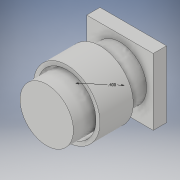
# Autodesk Inventor part: Ring Tolerance Test 6
Saved by Autodesk Inventor 2018 (Build 220112000, 112)
## iProperties
Created: 2019-08-26
Part Number: Ring Tolerance Test 6
Material: Generic
Document SubType Name: Modeling
Designer: 871357
Density: 1 g/cm^3
Appearance: Default
Author: 871357
Autodesk Inventor part; units mm, degrees
ref_plane "YZ Plane" through (0, 0, 0) normal (1, 0, 0) x (0, 1, 0)
ref_plane "XZ Plane" through (0, 0, 0) normal (0, 1, 0) x (-1, 0, 0)
ref_plane "XY Plane" through (0, 0, 0) normal (0, 0, 1) x (1, 0, 0)
sketch "Sketch1" plane through (0, 0, 0) normal (0, 0, 1) x (1, 0, 0)
  circle A0 centre (0, 0) radius 5.08
  dimension "d0" = 10.16
  constraints: 1 centre point, 1 coincident
  measures "d0" diameter of A0
extrude "Extrusion1" add sketch "Sketch1" along normal blind 10.16
ref_plane "Work Plane1" through (0, 0, 5.08) normal (0, 0, -1) x (-1, 0, 0)
sketch "Sketch4" plane through (0, 0, 0) normal (0, 0, -1) x (-1, 0, 0)
  circle A0 centre (0, 0) radius 5.588
  circle A1 centre (0, 0) radius 6.35
  dimension "d13" = 11.176
  dimension "d14" = 12.7
  constraints: 2 centre point, 2 coincident
  measures "d13" diameter of A0
  measures "d14" diameter of A1
extrude "Extrusion4" add sketch "Sketch4" against normal blind 6.35
extrude "Extrusion5" add sketch "Sketch1" against normal blind 3.81
sketch "Sketch5" plane through (0, 0, -3.81) normal (0, 0, -1) x (-1, 0, 0)
  line L0 (-6.35, -6.35) -> (6.35, -6.35)
  line L1 (6.35, -6.35) -> (6.35, 6.35)
  line L2 (6.35, 6.35) -> (-6.35, 6.35)
  line L3 (-6.35, 6.35) -> (-6.35, -6.35)
  point P0 (0, 0)
  dimension "d19" = 12.7
  dimension "d20" = 12.7
  dimension "d21" = 6.35
  dimension "d22" = 6.35
  constraints: 8 end point, 2 parallel, 1 horizontal, 1 perpendicular
  measures "d19" distance of L1.end L2.end
  measures "d20" distance of L0.end L1.end
  measures "d21" distance from line of point (0, 0) L2
  measures "d22" distance from line of L1 point (0, 0)
extrude "Extrusion6" add sketch "Sketch5" along normal blind 2.54
ref_plane "Work Plane2" through (0, 0, 3.175) normal (0, 0, 1) x (1, 0, 0)
body "Solid1"
